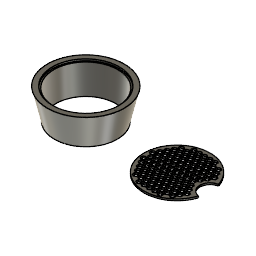
toyota-cup-holder (Autodesk Fusion 360 design; units mm, degrees)
part number: 2026-06-03-15-31-26-148
Autodesk Fusion 360 part; units mm, degrees
sketch "Sketch15" plane through (0, 0, 0) normal (0, 1, 0) x (1, 0, 0)
  line L0 (0, 0, 0) -> (0, 0, 40) construction
  line L1 (31, 0, 0) -> (37.8571, 0, 30)
  line L2 (37.8571, 0, 30) -> (32.8571, 0, 30)
  line L3 (32.8571, 0, 30) -> (32.8571, 0, 28.4)
  line L4 (32.8571, 0, 28.4) -> (31.4571, 0, 28.4)
  line L5 (31.4571, 0, 28.4) -> (29.8, 0, 0)
  line L6 (29.8, 0) -> (31, 0)
revolve "Revolve4" add sketch "Sketch15" angle 360 about axis through (0, 0, 0) along (0, 1, 0) contours L1 L2 L3 L4 L5 L6 in plane through (0, 0, 0) normal (0, 0, -1) makes body 1
move_body "Move1" bodies 1 to x (1, 0, 0) y (0, 0, 1) z (0, -1, 0) at (0, 0, 0)
sketch "Sketch16" plane through (0, 0, 0) normal (0, 0, 1) x (1, 0, 0)
  circle A0 centre (90, 0) radius 32.6
extrude "Extrude12" add sketch "Sketch16" along normal blind 1.6 separate body makes body 2
sketch "Sketch17" plane through (0, 0, 0) normal (0, 0, 1) x (1, 0, 0)
  circle A0 centre (122.6, 0) radius 10
extrude "Extrude13" cut sketch "Sketch17" along normal blind 1.6 bodies 2
sketch "HexGrid" plane through (0, 0, 0) normal (0, 0, 1) x (1, 0, 0)
  line L0 (81.6862, -25.8) -> (79.6077, -24.6)
  line L1 (79.6077, -24.6) -> (77.5292, -25.8)
  line L2 (77.5292, -25.8) -> (77.5292, -28.2)
  line L3 (77.5292, -28.2) -> (79.6077, -29.4)
  line L4 (79.6077, -29.4) -> (81.6862, -28.2)
  line L5 (81.6862, -28.2) -> (81.6862, -25.8)
  line L6 (86.8823, -25.8) -> (84.8038, -24.6)
  line L7 (84.8038, -24.6) -> (82.7254, -25.8)
  line L8 (82.7254, -25.8) -> (82.7254, -28.2)
  line L9 (82.7254, -28.2) -> (84.8038, -29.4)
  line L10 (84.8038, -29.4) -> (86.8823, -28.2)
  line L11 (86.8823, -28.2) -> (86.8823, -25.8)
  line L12 (92.0785, -25.8) -> (90, -24.6)
  line L13 (90, -24.6) -> (87.9215, -25.8)
  line L14 (87.9215, -25.8) -> (87.9215, -28.2)
  line L15 (87.9215, -28.2) -> (90, -29.4)
  line L16 (90, -29.4) -> (92.0785, -28.2)
  line L17 (92.0785, -28.2) -> (92.0785, -25.8)
  line L18 (97.2746, -25.8) -> (95.1962, -24.6)
  line L19 (95.1962, -24.6) -> (93.1177, -25.8)
  line L20 (93.1177, -25.8) -> (93.1177, -28.2)
  line L21 (93.1177, -28.2) -> (95.1962, -29.4)
  line L22 (95.1962, -29.4) -> (97.2746, -28.2)
  line L23 (97.2746, -28.2) -> (97.2746, -25.8)
  line L24 (102.4708, -25.8) -> (100.3923, -24.6)
  line L25 (100.3923, -24.6) -> (98.3138, -25.8)
  line L26 (98.3138, -25.8) -> (98.3138, -28.2)
  line L27 (98.3138, -28.2) -> (100.3923, -29.4)
  line L28 (100.3923, -29.4) -> (102.4708, -28.2)
  line L29 (102.4708, -28.2) -> (102.4708, -25.8)
  line L30 (73.8919, -21.3) -> (71.8135, -20.1)
  line L31 (71.8135, -20.1) -> (69.735, -21.3)
  line L32 (69.735, -21.3) -> (69.735, -23.7)
  line L33 (69.735, -23.7) -> (71.8135, -24.9)
  line L34 (71.8135, -24.9) -> (73.8919, -23.7)
  line L35 (73.8919, -23.7) -> (73.8919, -21.3)
  line L36 (79.0881, -21.3) -> (77.0096, -20.1)
  line L37 (77.0096, -20.1) -> (74.9312, -21.3)
  line L38 (74.9312, -21.3) -> (74.9312, -23.7)
  line L39 (74.9312, -23.7) -> (77.0096, -24.9)
  line L40 (77.0096, -24.9) -> (79.0881, -23.7)
  line L41 (79.0881, -23.7) -> (79.0881, -21.3)
  line L42 (84.2842, -21.3) -> (82.2058, -20.1)
  line L43 (82.2058, -20.1) -> (80.1273, -21.3)
  line L44 (80.1273, -21.3) -> (80.1273, -23.7)
  line L45 (80.1273, -23.7) -> (82.2058, -24.9)
  line L46 (82.2058, -24.9) -> (84.2842, -23.7)
  line L47 (84.2842, -23.7) -> (84.2842, -21.3)
  line L48 (89.4804, -21.3) -> (87.4019, -20.1)
  line L49 (87.4019, -20.1) -> (85.3235, -21.3)
  line L50 (85.3235, -21.3) -> (85.3235, -23.7)
  line L51 (85.3235, -23.7) -> (87.4019, -24.9)
  line L52 (87.4019, -24.9) -> (89.4804, -23.7)
  line L53 (89.4804, -23.7) -> (89.4804, -21.3)
  line L54 (94.6765, -21.3) -> (92.5981, -20.1)
  line L55 (92.5981, -20.1) -> (90.5196, -21.3)
  line L56 (90.5196, -21.3) -> (90.5196, -23.7)
  line L57 (90.5196, -23.7) -> (92.5981, -24.9)
  line L58 (92.5981, -24.9) -> (94.6765, -23.7)
  line L59 (94.6765, -23.7) -> (94.6765, -21.3)
  line L60 (99.8727, -21.3) -> (97.7942, -20.1)
  line L61 (97.7942, -20.1) -> (95.7158, -21.3)
  line L62 (95.7158, -21.3) -> (95.7158, -23.7)
  line L63 (95.7158, -23.7) -> (97.7942, -24.9)
  line L64 (97.7942, -24.9) -> (99.8727, -23.7)
  line L65 (99.8727, -23.7) -> (99.8727, -21.3)
  line L66 (105.0688, -21.3) -> (102.9904, -20.1)
  line L67 (102.9904, -20.1) -> (100.9119, -21.3)
  line L68 (100.9119, -21.3) -> (100.9119, -23.7)
  line L69 (100.9119, -23.7) -> (102.9904, -24.9)
  line L70 (102.9904, -24.9) -> (105.0688, -23.7)
  line L71 (105.0688, -23.7) -> (105.0688, -21.3)
  line L72 (110.265, -21.3) -> (108.1865, -20.1)
  line L73 (108.1865, -20.1) -> (106.1081, -21.3)
  line L74 (106.1081, -21.3) -> (106.1081, -23.7)
  line L75 (106.1081, -23.7) -> (108.1865, -24.9)
  line L76 (108.1865, -24.9) -> (110.265, -23.7)
  line L77 (110.265, -23.7) -> (110.265, -21.3)
  line L78 (71.2939, -16.8) -> (69.2154, -15.6)
  line L79 (69.2154, -15.6) -> (67.1369, -16.8)
  line L80 (67.1369, -16.8) -> (67.1369, -19.2)
  line L81 (67.1369, -19.2) -> (69.2154, -20.4)
  line L82 (69.2154, -20.4) -> (71.2939, -19.2)
  line L83 (71.2939, -19.2) -> (71.2939, -16.8)
  line L84 (76.49, -16.8) -> (74.4115, -15.6)
  line L85 (74.4115, -15.6) -> (72.3331, -16.8)
  line L86 (72.3331, -16.8) -> (72.3331, -19.2)
  line L87 (72.3331, -19.2) -> (74.4115, -20.4)
  line L88 (74.4115, -20.4) -> (76.49, -19.2)
  line L89 (76.49, -19.2) -> (76.49, -16.8)
  line L90 (81.6862, -16.8) -> (79.6077, -15.6)
  line L91 (79.6077, -15.6) -> (77.5292, -16.8)
  line L92 (77.5292, -16.8) -> (77.5292, -19.2)
  line L93 (77.5292, -19.2) -> (79.6077, -20.4)
  line L94 (79.6077, -20.4) -> (81.6862, -19.2)
  line L95 (81.6862, -19.2) -> (81.6862, -16.8)
  line L96 (86.8823, -16.8) -> (84.8038, -15.6)
  line L97 (84.8038, -15.6) -> (82.7254, -16.8)
  line L98 (82.7254, -16.8) -> (82.7254, -19.2)
  line L99 (82.7254, -19.2) -> (84.8038, -20.4)
  line L100 (84.8038, -20.4) -> (86.8823, -19.2)
  line L101 (86.8823, -19.2) -> (86.8823, -16.8)
  line L102 (92.0785, -16.8) -> (90, -15.6)
  line L103 (90, -15.6) -> (87.9215, -16.8)
  line L104 (87.9215, -16.8) -> (87.9215, -19.2)
  line L105 (87.9215, -19.2) -> (90, -20.4)
  line L106 (90, -20.4) -> (92.0785, -19.2)
  line L107 (92.0785, -19.2) -> (92.0785, -16.8)
  line L108 (97.2746, -16.8) -> (95.1962, -15.6)
  line L109 (95.1962, -15.6) -> (93.1177, -16.8)
  line L110 (93.1177, -16.8) -> (93.1177, -19.2)
  line L111 (93.1177, -19.2) -> (95.1962, -20.4)
  line L112 (95.1962, -20.4) -> (97.2746, -19.2)
  line L113 (97.2746, -19.2) -> (97.2746, -16.8)
  line L114 (102.4708, -16.8) -> (100.3923, -15.6)
  line L115 (100.3923, -15.6) -> (98.3138, -16.8)
  line L116 (98.3138, -16.8) -> (98.3138, -19.2)
  line L117 (98.3138, -19.2) -> (100.3923, -20.4)
  line L118 (100.3923, -20.4) -> (102.4708, -19.2)
  line L119 (102.4708, -19.2) -> (102.4708, -16.8)
  line L120 (107.6669, -16.8) -> (105.5885, -15.6)
  line L121 (105.5885, -15.6) -> (103.51, -16.8)
  line L122 (103.51, -16.8) -> (103.51, -19.2)
  line L123 (103.51, -19.2) -> (105.5885, -20.4)
  line L124 (105.5885, -20.4) -> (107.6669, -19.2)
  line L125 (107.6669, -19.2) -> (107.6669, -16.8)
  line L126 (112.8631, -16.8) -> (110.7846, -15.6)
  line L127 (110.7846, -15.6) -> (108.7061, -16.8)
  line L128 (108.7061, -16.8) -> (108.7061, -19.2)
  line L129 (108.7061, -19.2) -> (110.7846, -20.4)
  line L130 (110.7846, -20.4) -> (112.8631, -19.2)
  line L131 (112.8631, -19.2) -> (112.8631, -16.8)
  line L132 (68.6958, -12.3) -> (66.6173, -11.1)
  line L133 (66.6173, -11.1) -> (64.5389, -12.3)
  line L134 (64.5389, -12.3) -> (64.5389, -14.7)
  line L135 (64.5389, -14.7) -> (66.6173, -15.9)
  line L136 (66.6173, -15.9) -> (68.6958, -14.7)
  line L137 (68.6958, -14.7) -> (68.6958, -12.3)
  line L138 (73.8919, -12.3) -> (71.8135, -11.1)
  line L139 (71.8135, -11.1) -> (69.735, -12.3)
  line L140 (69.735, -12.3) -> (69.735, -14.7)
  line L141 (69.735, -14.7) -> (71.8135, -15.9)
  line L142 (71.8135, -15.9) -> (73.8919, -14.7)
  line L143 (73.8919, -14.7) -> (73.8919, -12.3)
  line L144 (79.0881, -12.3) -> (77.0096, -11.1)
  line L145 (77.0096, -11.1) -> (74.9312, -12.3)
  line L146 (74.9312, -12.3) -> (74.9312, -14.7)
  line L147 (74.9312, -14.7) -> (77.0096, -15.9)
  line L148 (77.0096, -15.9) -> (79.0881, -14.7)
  line L149 (79.0881, -14.7) -> (79.0881, -12.3)
  line L150 (84.2842, -12.3) -> (82.2058, -11.1)
  line L151 (82.2058, -11.1) -> (80.1273, -12.3)
  line L152 (80.1273, -12.3) -> (80.1273, -14.7)
  line L153 (80.1273, -14.7) -> (82.2058, -15.9)
  line L154 (82.2058, -15.9) -> (84.2842, -14.7)
  line L155 (84.2842, -14.7) -> (84.2842, -12.3)
  line L156 (89.4804, -12.3) -> (87.4019, -11.1)
  line L157 (87.4019, -11.1) -> (85.3235, -12.3)
  line L158 (85.3235, -12.3) -> (85.3235, -14.7)
  line L159 (85.3235, -14.7) -> (87.4019, -15.9)
  line L160 (87.4019, -15.9) -> (89.4804, -14.7)
  line L161 (89.4804, -14.7) -> (89.4804, -12.3)
  line L162 (94.6765, -12.3) -> (92.5981, -11.1)
  line L163 (92.5981, -11.1) -> (90.5196, -12.3)
  line L164 (90.5196, -12.3) -> (90.5196, -14.7)
  line L165 (90.5196, -14.7) -> (92.5981, -15.9)
  line L166 (92.5981, -15.9) -> (94.6765, -14.7)
  line L167 (94.6765, -14.7) -> (94.6765, -12.3)
  line L168 (99.8727, -12.3) -> (97.7942, -11.1)
  line L169 (97.7942, -11.1) -> (95.7158, -12.3)
  line L170 (95.7158, -12.3) -> (95.7158, -14.7)
  line L171 (95.7158, -14.7) -> (97.7942, -15.9)
  line L172 (97.7942, -15.9) -> (99.8727, -14.7)
  line L173 (99.8727, -14.7) -> (99.8727, -12.3)
  line L174 (105.0688, -12.3) -> (102.9904, -11.1)
  line L175 (102.9904, -11.1) -> (100.9119, -12.3)
  line L176 (100.9119, -12.3) -> (100.9119, -14.7)
  line L177 (100.9119, -14.7) -> (102.9904, -15.9)
  line L178 (102.9904, -15.9) -> (105.0688, -14.7)
  line L179 (105.0688, -14.7) -> (105.0688, -12.3)
  line L180 (110.265, -12.3) -> (108.1865, -11.1)
  line L181 (108.1865, -11.1) -> (106.1081, -12.3)
  line L182 (106.1081, -12.3) -> (106.1081, -14.7)
  line L183 (106.1081, -14.7) -> (108.1865, -15.9)
  line L184 (108.1865, -15.9) -> (110.265, -14.7)
  line L185 (110.265, -14.7) -> (110.265, -12.3)
  line L186 (115.4611, -12.3) -> (113.3827, -11.1)
  line L187 (113.3827, -11.1) -> (111.3042, -12.3)
  line L188 (111.3042, -12.3) -> (111.3042, -14.7)
  line L189 (111.3042, -14.7) -> (113.3827, -15.9)
  line L190 (113.3827, -15.9) -> (115.4611, -14.7)
  line L191 (115.4611, -14.7) -> (115.4611, -12.3)
  line L192 (66.0977, -7.8) -> (64.0192, -6.6)
  line L193 (64.0192, -6.6) -> (61.9408, -7.8)
  line L194 (61.9408, -7.8) -> (61.9408, -10.2)
  line L195 (61.9408, -10.2) -> (64.0192, -11.4)
  line L196 (64.0192, -11.4) -> (66.0977, -10.2)
  line L197 (66.0977, -10.2) -> (66.0977, -7.8)
  line L198 (71.2939, -7.8) -> (69.2154, -6.6)
  line L199 (69.2154, -6.6) -> (67.1369, -7.8)
  line L200 (67.1369, -7.8) -> (67.1369, -10.2)
  line L201 (67.1369, -10.2) -> (69.2154, -11.4)
  line L202 (69.2154, -11.4) -> (71.2939, -10.2)
  line L203 (71.2939, -10.2) -> (71.2939, -7.8)
  line L204 (76.49, -7.8) -> (74.4115, -6.6)
  line L205 (74.4115, -6.6) -> (72.3331, -7.8)
  line L206 (72.3331, -7.8) -> (72.3331, -10.2)
  line L207 (72.3331, -10.2) -> (74.4115, -11.4)
  line L208 (74.4115, -11.4) -> (76.49, -10.2)
  line L209 (76.49, -10.2) -> (76.49, -7.8)
  line L210 (81.6862, -7.8) -> (79.6077, -6.6)
  line L211 (79.6077, -6.6) -> (77.5292, -7.8)
  line L212 (77.5292, -7.8) -> (77.5292, -10.2)
  line L213 (77.5292, -10.2) -> (79.6077, -11.4)
  line L214 (79.6077, -11.4) -> (81.6862, -10.2)
  line L215 (81.6862, -10.2) -> (81.6862, -7.8)
  line L216 (86.8823, -7.8) -> (84.8038, -6.6)
  line L217 (84.8038, -6.6) -> (82.7254, -7.8)
  line L218 (82.7254, -7.8) -> (82.7254, -10.2)
  line L219 (82.7254, -10.2) -> (84.8038, -11.4)
  line L220 (84.8038, -11.4) -> (86.8823, -10.2)
  line L221 (86.8823, -10.2) -> (86.8823, -7.8)
  line L222 (92.0785, -7.8) -> (90, -6.6)
  line L223 (90, -6.6) -> (87.9215, -7.8)
  line L224 (87.9215, -7.8) -> (87.9215, -10.2)
  line L225 (87.9215, -10.2) -> (90, -11.4)
  line L226 (90, -11.4) -> (92.0785, -10.2)
  line L227 (92.0785, -10.2) -> (92.0785, -7.8)
  line L228 (97.2746, -7.8) -> (95.1962, -6.6)
  line L229 (95.1962, -6.6) -> (93.1177, -7.8)
  line L230 (93.1177, -7.8) -> (93.1177, -10.2)
  line L231 (93.1177, -10.2) -> (95.1962, -11.4)
  line L232 (95.1962, -11.4) -> (97.2746, -10.2)
  line L233 (97.2746, -10.2) -> (97.2746, -7.8)
  line L234 (102.4708, -7.8) -> (100.3923, -6.6)
  line L235 (100.3923, -6.6) -> (98.3138, -7.8)
  line L236 (98.3138, -7.8) -> (98.3138, -10.2)
  line L237 (98.3138, -10.2) -> (100.3923, -11.4)
  line L238 (100.3923, -11.4) -> (102.4708, -10.2)
  line L239 (102.4708, -10.2) -> (102.4708, -7.8)
  line L240 (107.6669, -7.8) -> (105.5885, -6.6)
  line L241 (105.5885, -6.6) -> (103.51, -7.8)
  line L242 (103.51, -7.8) -> (103.51, -10.2)
  line L243 (103.51, -10.2) -> (105.5885, -11.4)
  line L244 (105.5885, -11.4) -> (107.6669, -10.2)
  line L245 (107.6669, -10.2) -> (107.6669, -7.8)
  line L246 (112.8631, -7.8) -> (110.7846, -6.6)
  line L247 (110.7846, -6.6) -> (108.7061, -7.8)
  line L248 (108.7061, -7.8) -> (108.7061, -10.2)
  line L249 (108.7061, -10.2) -> (110.7846, -11.4)
  line L250 (110.7846, -11.4) -> (112.8631, -10.2)
  line L251 (112.8631, -10.2) -> (112.8631, -7.8)
  line L252 (63.4996, -3.3) -> (61.4212, -2.1)
  line L253 (61.4212, -2.1) -> (59.3427, -3.3)
  line L254 (59.3427, -3.3) -> (59.3427, -5.7)
  line L255 (59.3427, -5.7) -> (61.4212, -6.9)
  line L256 (61.4212, -6.9) -> (63.4996, -5.7)
  line L257 (63.4996, -5.7) -> (63.4996, -3.3)
  line L258 (68.6958, -3.3) -> (66.6173, -2.1)
  line L259 (66.6173, -2.1) -> (64.5389, -3.3)
  line L260 (64.5389, -3.3) -> (64.5389, -5.7)
  line L261 (64.5389, -5.7) -> (66.6173, -6.9)
  line L262 (66.6173, -6.9) -> (68.6958, -5.7)
  line L263 (68.6958, -5.7) -> (68.6958, -3.3)
  line L264 (73.8919, -3.3) -> (71.8135, -2.1)
  line L265 (71.8135, -2.1) -> (69.735, -3.3)
  line L266 (69.735, -3.3) -> (69.735, -5.7)
  line L267 (69.735, -5.7) -> (71.8135, -6.9)
  line L268 (71.8135, -6.9) -> (73.8919, -5.7)
  line L269 (73.8919, -5.7) -> (73.8919, -3.3)
  line L270 (79.0881, -3.3) -> (77.0096, -2.1)
  line L271 (77.0096, -2.1) -> (74.9312, -3.3)
  line L272 (74.9312, -3.3) -> (74.9312, -5.7)
  line L273 (74.9312, -5.7) -> (77.0096, -6.9)
  line L274 (77.0096, -6.9) -> (79.0881, -5.7)
  line L275 (79.0881, -5.7) -> (79.0881, -3.3)
  line L276 (84.2842, -3.3) -> (82.2058, -2.1)
  line L277 (82.2058, -2.1) -> (80.1273, -3.3)
  line L278 (80.1273, -3.3) -> (80.1273, -5.7)
  line L279 (80.1273, -5.7) -> (82.2058, -6.9)
  line L280 (82.2058, -6.9) -> (84.2842, -5.7)
  line L281 (84.2842, -5.7) -> (84.2842, -3.3)
  line L282 (89.4804, -3.3) -> (87.4019, -2.1)
  line L283 (87.4019, -2.1) -> (85.3235, -3.3)
  line L284 (85.3235, -3.3) -> (85.3235, -5.7)
  line L285 (85.3235, -5.7) -> (87.4019, -6.9)
  line L286 (87.4019, -6.9) -> (89.4804, -5.7)
  line L287 (89.4804, -5.7) -> (89.4804, -3.3)
  line L288 (94.6765, -3.3) -> (92.5981, -2.1)
  line L289 (92.5981, -2.1) -> (90.5196, -3.3)
  line L290 (90.5196, -3.3) -> (90.5196, -5.7)
  line L291 (90.5196, -5.7) -> (92.5981, -6.9)
  line L292 (92.5981, -6.9) -> (94.6765, -5.7)
  line L293 (94.6765, -5.7) -> (94.6765, -3.3)
  line L294 (99.8727, -3.3) -> (97.7942, -2.1)
  line L295 (97.7942, -2.1) -> (95.7158, -3.3)
  line L296 (95.7158, -3.3) -> (95.7158, -5.7)
  line L297 (95.7158, -5.7) -> (97.7942, -6.9)
  line L298 (97.7942, -6.9) -> (99.8727, -5.7)
  line L299 (99.8727, -5.7) -> (99.8727, -3.3)
  line L300 (105.0688, -3.3) -> (102.9904, -2.1)
  line L301 (102.9904, -2.1) -> (100.9119, -3.3)
  line L302 (100.9119, -3.3) -> (100.9119, -5.7)
  line L303 (100.9119, -5.7) -> (102.9904, -6.9)
  line L304 (102.9904, -6.9) -> (105.0688, -5.7)
  line L305 (105.0688, -5.7) -> (105.0688, -3.3)
  line L306 (110.265, -3.3) -> (108.1865, -2.1)
  line L307 (108.1865, -2.1) -> (106.1081, -3.3)
  line L308 (106.1081, -3.3) -> (106.1081, -5.7)
  line L309 (106.1081, -5.7) -> (108.1865, -6.9)
  line L310 (108.1865, -6.9) -> (110.265, -5.7)
  line L311 (110.265, -5.7) -> (110.265, -3.3)
  line L312 (66.0977, 1.2) -> (64.0192, 2.4)
  line L313 (64.0192, 2.4) -> (61.9408, 1.2)
  line L314 (61.9408, 1.2) -> (61.9408, -1.2)
  line L315 (61.9408, -1.2) -> (64.0192, -2.4)
  line L316 (64.0192, -2.4) -> (66.0977, -1.2)
  line L317 (66.0977, -1.2) -> (66.0977, 1.2)
  line L318 (71.2939, 1.2) -> (69.2154, 2.4)
  line L319 (69.2154, 2.4) -> (67.1369, 1.2)
  line L320 (67.1369, 1.2) -> (67.1369, -1.2)
  line L321 (67.1369, -1.2) -> (69.2154, -2.4)
  line L322 (69.2154, -2.4) -> (71.2939, -1.2)
  line L323 (71.2939, -1.2) -> (71.2939, 1.2)
  line L324 (76.49, 1.2) -> (74.4115, 2.4)
  line L325 (74.4115, 2.4) -> (72.3331, 1.2)
  line L326 (72.3331, 1.2) -> (72.3331, -1.2)
  line L327 (72.3331, -1.2) -> (74.4115, -2.4)
  line L328 (74.4115, -2.4) -> (76.49, -1.2)
  line L329 (76.49, -1.2) -> (76.49, 1.2)
  line L330 (81.6862, 1.2) -> (79.6077, 2.4)
  line L331 (79.6077, 2.4) -> (77.5292, 1.2)
  line L332 (77.5292, 1.2) -> (77.5292, -1.2)
  line L333 (77.5292, -1.2) -> (79.6077, -2.4)
  line L334 (79.6077, -2.4) -> (81.6862, -1.2)
  line L335 (81.6862, -1.2) -> (81.6862, 1.2)
  line L336 (86.8823, 1.2) -> (84.8038, 2.4)
  line L337 (84.8038, 2.4) -> (82.7254, 1.2)
  line L338 (82.7254, 1.2) -> (82.7254, -1.2)
  line L339 (82.7254, -1.2) -> (84.8038, -2.4)
  line L340 (84.8038, -2.4) -> (86.8823, -1.2)
  line L341 (86.8823, -1.2) -> (86.8823, 1.2)
  line L342 (92.0785, 1.2) -> (90, 2.4)
  line L343 (90, 2.4) -> (87.9215, 1.2)
  line L344 (87.9215, 1.2) -> (87.9215, -1.2)
  line L345 (87.9215, -1.2) -> (90, -2.4)
  line L346 (90, -2.4) -> (92.0785, -1.2)
  line L347 (92.0785, -1.2) -> (92.0785, 1.2)
  line L348 (97.2746, 1.2) -> (95.1962, 2.4)
  line L349 (95.1962, 2.4) -> (93.1177, 1.2)
  line L350 (93.1177, 1.2) -> (93.1177, -1.2)
  line L351 (93.1177, -1.2) -> (95.1962, -2.4)
  line L352 (95.1962, -2.4) -> (97.2746, -1.2)
  line L353 (97.2746, -1.2) -> (97.2746, 1.2)
  line L354 (102.4708, 1.2) -> (100.3923, 2.4)
  line L355 (100.3923, 2.4) -> (98.3138, 1.2)
  line L356 (98.3138, 1.2) -> (98.3138, -1.2)
  line L357 (98.3138, -1.2) -> (100.3923, -2.4)
  line L358 (100.3923, -2.4) -> (102.4708, -1.2)
  line L359 (102.4708, -1.2) -> (102.4708, 1.2)
  line L360 (107.6669, 1.2) -> (105.5885, 2.4)
  line L361 (105.5885, 2.4) -> (103.51, 1.2)
  line L362 (103.51, 1.2) -> (103.51, -1.2)
  line L363 (103.51, -1.2) -> (105.5885, -2.4)
  line L364 (105.5885, -2.4) -> (107.6669, -1.2)
  line L365 (107.6669, -1.2) -> (107.6669, 1.2)
  line L366 (63.4996, 5.7) -> (61.4212, 6.9)
  line L367 (61.4212, 6.9) -> (59.3427, 5.7)
  line L368 (59.3427, 5.7) -> (59.3427, 3.3)
  line L369 (59.3427, 3.3) -> (61.4212, 2.1)
  line L370 (61.4212, 2.1) -> (63.4996, 3.3)
  line L371 (63.4996, 3.3) -> (63.4996, 5.7)
  line L372 (68.6958, 5.7) -> (66.6173, 6.9)
  line L373 (66.6173, 6.9) -> (64.5389, 5.7)
  line L374 (64.5389, 5.7) -> (64.5389, 3.3)
  line L375 (64.5389, 3.3) -> (66.6173, 2.1)
  line L376 (66.6173, 2.1) -> (68.6958, 3.3)
  line L377 (68.6958, 3.3) -> (68.6958, 5.7)
  line L378 (73.8919, 5.7) -> (71.8135, 6.9)
  line L379 (71.8135, 6.9) -> (69.735, 5.7)
  line L380 (69.735, 5.7) -> (69.735, 3.3)
  line L381 (69.735, 3.3) -> (71.8135, 2.1)
  line L382 (71.8135, 2.1) -> (73.8919, 3.3)
  line L383 (73.8919, 3.3) -> (73.8919, 5.7)
  line L384 (79.0881, 5.7) -> (77.0096, 6.9)
  line L385 (77.0096, 6.9) -> (74.9312, 5.7)
  line L386 (74.9312, 5.7) -> (74.9312, 3.3)
  line L387 (74.9312, 3.3) -> (77.0096, 2.1)
  line L388 (77.0096, 2.1) -> (79.0881, 3.3)
  line L389 (79.0881, 3.3) -> (79.0881, 5.7)
  line L390 (84.2842, 5.7) -> (82.2058, 6.9)
  line L391 (82.2058, 6.9) -> (80.1273, 5.7)
  line L392 (80.1273, 5.7) -> (80.1273, 3.3)
  line L393 (80.1273, 3.3) -> (82.2058, 2.1)
  line L394 (82.2058, 2.1) -> (84.2842, 3.3)
  line L395 (84.2842, 3.3) -> (84.2842, 5.7)
  line L396 (89.4804, 5.7) -> (87.4019, 6.9)
  line L397 (87.4019, 6.9) -> (85.3235, 5.7)
  line L398 (85.3235, 5.7) -> (85.3235, 3.3)
  line L399 (85.3235, 3.3) -> (87.4019, 2.1)
  line L400 (87.4019, 2.1) -> (89.4804, 3.3)
  line L401 (89.4804, 3.3) -> (89.4804, 5.7)
  line L402 (94.6765, 5.7) -> (92.5981, 6.9)
  line L403 (92.5981, 6.9) -> (90.5196, 5.7)
  line L404 (90.5196, 5.7) -> (90.5196, 3.3)
  line L405 (90.5196, 3.3) -> (92.5981, 2.1)
  line L406 (92.5981, 2.1) -> (94.6765, 3.3)
  line L407 (94.6765, 3.3) -> (94.6765, 5.7)
  line L408 (99.8727, 5.7) -> (97.7942, 6.9)
  line L409 (97.7942, 6.9) -> (95.7158, 5.7)
  line L410 (95.7158, 5.7) -> (95.7158, 3.3)
  line L411 (95.7158, 3.3) -> (97.7942, 2.1)
  line L412 (97.7942, 2.1) -> (99.8727, 3.3)
  line L413 (99.8727, 3.3) -> (99.8727, 5.7)
  line L414 (105.0688, 5.7) -> (102.9904, 6.9)
  line L415 (102.9904, 6.9) -> (100.9119, 5.7)
  line L416 (100.9119, 5.7) -> (100.9119, 3.3)
  line L417 (100.9119, 3.3) -> (102.9904, 2.1)
  line L418 (102.9904, 2.1) -> (105.0688, 3.3)
  line L419 (105.0688, 3.3) -> (105.0688, 5.7)
  line L420 (110.265, 5.7) -> (108.1865, 6.9)
  line L421 (108.1865, 6.9) -> (106.1081, 5.7)
  line L422 (106.1081, 5.7) -> (106.1081, 3.3)
  line L423 (106.1081, 3.3) -> (108.1865, 2.1)
  line L424 (108.1865, 2.1) -> (110.265, 3.3)
  line L425 (110.265, 3.3) -> (110.265, 5.7)
  line L426 (66.0977, 10.2) -> (64.0192, 11.4)
  line L427 (64.0192, 11.4) -> (61.9408, 10.2)
  line L428 (61.9408, 10.2) -> (61.9408, 7.8)
  line L429 (61.9408, 7.8) -> (64.0192, 6.6)
  line L430 (64.0192, 6.6) -> (66.0977, 7.8)
  line L431 (66.0977, 7.8) -> (66.0977, 10.2)
  line L432 (71.2939, 10.2) -> (69.2154, 11.4)
  line L433 (69.2154, 11.4) -> (67.1369, 10.2)
  line L434 (67.1369, 10.2) -> (67.1369, 7.8)
  line L435 (67.1369, 7.8) -> (69.2154, 6.6)
  line L436 (69.2154, 6.6) -> (71.2939, 7.8)
  line L437 (71.2939, 7.8) -> (71.2939, 10.2)
  line L438 (76.49, 10.2) -> (74.4115, 11.4)
  line L439 (74.4115, 11.4) -> (72.3331, 10.2)
  line L440 (72.3331, 10.2) -> (72.3331, 7.8)
  line L441 (72.3331, 7.8) -> (74.4115, 6.6)
  line L442 (74.4115, 6.6) -> (76.49, 7.8)
  line L443 (76.49, 7.8) -> (76.49, 10.2)
  line L444 (81.6862, 10.2) -> (79.6077, 11.4)
  line L445 (79.6077, 11.4) -> (77.5292, 10.2)
  line L446 (77.5292, 10.2) -> (77.5292, 7.8)
  line L447 (77.5292, 7.8) -> (79.6077, 6.6)
  line L448 (79.6077, 6.6) -> (81.6862, 7.8)
  line L449 (81.6862, 7.8) -> (81.6862, 10.2)
  line L450 (86.8823, 10.2) -> (84.8038, 11.4)
  line L451 (84.8038, 11.4) -> (82.7254, 10.2)
  line L452 (82.7254, 10.2) -> (82.7254, 7.8)
  line L453 (82.7254, 7.8) -> (84.8038, 6.6)
  line L454 (84.8038, 6.6) -> (86.8823, 7.8)
  line L455 (86.8823, 7.8) -> (86.8823, 10.2)
  line L456 (92.0785, 10.2) -> (90, 11.4)
  line L457 (90, 11.4) -> (87.9215, 10.2)
  line L458 (87.9215, 10.2) -> (87.9215, 7.8)
  line L459 (87.9215, 7.8) -> (90, 6.6)
  line L460 (90, 6.6) -> (92.0785, 7.8)
  line L461 (92.0785, 7.8) -> (92.0785, 10.2)
  line L462 (97.2746, 10.2) -> (95.1962, 11.4)
  line L463 (95.1962, 11.4) -> (93.1177, 10.2)
  line L464 (93.1177, 10.2) -> (93.1177, 7.8)
  line L465 (93.1177, 7.8) -> (95.1962, 6.6)
  line L466 (95.1962, 6.6) -> (97.2746, 7.8)
  line L467 (97.2746, 7.8) -> (97.2746, 10.2)
  line L468 (102.4708, 10.2) -> (100.3923, 11.4)
  line L469 (100.3923, 11.4) -> (98.3138, 10.2)
  line L470 (98.3138, 10.2) -> (98.3138, 7.8)
  line L471 (98.3138, 7.8) -> (100.3923, 6.6)
  line L472 (100.3923, 6.6) -> (102.4708, 7.8)
  line L473 (102.4708, 7.8) -> (102.4708, 10.2)
  line L474 (107.6669, 10.2) -> (105.5885, 11.4)
  line L475 (105.5885, 11.4) -> (103.51, 10.2)
  line L476 (103.51, 10.2) -> (103.51, 7.8)
  line L477 (103.51, 7.8) -> (105.5885, 6.6)
  line L478 (105.5885, 6.6) -> (107.6669, 7.8)
  line L479 (107.6669, 7.8) -> (107.6669, 10.2)
  line L480 (112.8631, 10.2) -> (110.7846, 11.4)
  line L481 (110.7846, 11.4) -> (108.7061, 10.2)
  line L482 (108.7061, 10.2) -> (108.7061, 7.8)
  line L483 (108.7061, 7.8) -> (110.7846, 6.6)
  line L484 (110.7846, 6.6) -> (112.8631, 7.8)
  line L485 (112.8631, 7.8) -> (112.8631, 10.2)
  line L486 (68.6958, 14.7) -> (66.6173, 15.9)
  line L487 (66.6173, 15.9) -> (64.5389, 14.7)
  line L488 (64.5389, 14.7) -> (64.5389, 12.3)
  line L489 (64.5389, 12.3) -> (66.6173, 11.1)
  line L490 (66.6173, 11.1) -> (68.6958, 12.3)
  line L491 (68.6958, 12.3) -> (68.6958, 14.7)
  line L492 (73.8919, 14.7) -> (71.8135, 15.9)
  line L493 (71.8135, 15.9) -> (69.735, 14.7)
  line L494 (69.735, 14.7) -> (69.735, 12.3)
  line L495 (69.735, 12.3) -> (71.8135, 11.1)
  line L496 (71.8135, 11.1) -> (73.8919, 12.3)
  line L497 (73.8919, 12.3) -> (73.8919, 14.7)
  line L498 (79.0881, 14.7) -> (77.0096, 15.9)
  line L499 (77.0096, 15.9) -> (74.9312, 14.7)
  line L500 (74.9312, 14.7) -> (74.9312, 12.3)
  line L501 (74.9312, 12.3) -> (77.0096, 11.1)
  line L502 (77.0096, 11.1) -> (79.0881, 12.3)
  line L503 (79.0881, 12.3) -> (79.0881, 14.7)
  line L504 (84.2842, 14.7) -> (82.2058, 15.9)
  line L505 (82.2058, 15.9) -> (80.1273, 14.7)
  line L506 (80.1273, 14.7) -> (80.1273, 12.3)
  line L507 (80.1273, 12.3) -> (82.2058, 11.1)
  line L508 (82.2058, 11.1) -> (84.2842, 12.3)
  line L509 (84.2842, 12.3) -> (84.2842, 14.7)
  line L510 (89.4804, 14.7) -> (87.4019, 15.9)
  line L511 (87.4019, 15.9) -> (85.3235, 14.7)
  line L512 (85.3235, 14.7) -> (85.3235, 12.3)
  line L513 (85.3235, 12.3) -> (87.4019, 11.1)
  line L514 (87.4019, 11.1) -> (89.4804, 12.3)
  line L515 (89.4804, 12.3) -> (89.4804, 14.7)
  line L516 (94.6765, 14.7) -> (92.5981, 15.9)
  line L517 (92.5981, 15.9) -> (90.5196, 14.7)
  line L518 (90.5196, 14.7) -> (90.5196, 12.3)
  line L519 (90.5196, 12.3) -> (92.5981, 11.1)
  line L520 (92.5981, 11.1) -> (94.6765, 12.3)
  line L521 (94.6765, 12.3) -> (94.6765, 14.7)
  line L522 (99.8727, 14.7) -> (97.7942, 15.9)
  line L523 (97.7942, 15.9) -> (95.7158, 14.7)
  line L524 (95.7158, 14.7) -> (95.7158, 12.3)
  line L525 (95.7158, 12.3) -> (97.7942, 11.1)
  line L526 (97.7942, 11.1) -> (99.8727, 12.3)
  line L527 (99.8727, 12.3) -> (99.8727, 14.7)
  line L528 (105.0688, 14.7) -> (102.9904, 15.9)
  line L529 (102.9904, 15.9) -> (100.9119, 14.7)
  line L530 (100.9119, 14.7) -> (100.9119, 12.3)
  line L531 (100.9119, 12.3) -> (102.9904, 11.1)
  line L532 (102.9904, 11.1) -> (105.0688, 12.3)
  line L533 (105.0688, 12.3) -> (105.0688, 14.7)
  line L534 (110.265, 14.7) -> (108.1865, 15.9)
  line L535 (108.1865, 15.9) -> (106.1081, 14.7)
  line L536 (106.1081, 14.7) -> (106.1081, 12.3)
  line L537 (106.1081, 12.3) -> (108.1865, 11.1)
  line L538 (108.1865, 11.1) -> (110.265, 12.3)
  line L539 (110.265, 12.3) -> (110.265, 14.7)
  line L540 (115.4611, 14.7) -> (113.3827, 15.9)
  line L541 (113.3827, 15.9) -> (111.3042, 14.7)
  line L542 (111.3042, 14.7) -> (111.3042, 12.3)
  line L543 (111.3042, 12.3) -> (113.3827, 11.1)
  line L544 (113.3827, 11.1) -> (115.4611, 12.3)
  line L545 (115.4611, 12.3) -> (115.4611, 14.7)
  line L546 (71.2939, 19.2) -> (69.2154, 20.4)
  line L547 (69.2154, 20.4) -> (67.1369, 19.2)
  line L548 (67.1369, 19.2) -> (67.1369, 16.8)
  line L549 (67.1369, 16.8) -> (69.2154, 15.6)
  line L550 (69.2154, 15.6) -> (71.2939, 16.8)
  line L551 (71.2939, 16.8) -> (71.2939, 19.2)
  line L552 (76.49, 19.2) -> (74.4115, 20.4)
  line L553 (74.4115, 20.4) -> (72.3331, 19.2)
  line L554 (72.3331, 19.2) -> (72.3331, 16.8)
  line L555 (72.3331, 16.8) -> (74.4115, 15.6)
  line L556 (74.4115, 15.6) -> (76.49, 16.8)
  line L557 (76.49, 16.8) -> (76.49, 19.2)
  line L558 (81.6862, 19.2) -> (79.6077, 20.4)
  line L559 (79.6077, 20.4) -> (77.5292, 19.2)
  line L560 (77.5292, 19.2) -> (77.5292, 16.8)
  line L561 (77.5292, 16.8) -> (79.6077, 15.6)
  line L562 (79.6077, 15.6) -> (81.6862, 16.8)
  line L563 (81.6862, 16.8) -> (81.6862, 19.2)
  line L564 (86.8823, 19.2) -> (84.8038, 20.4)
  line L565 (84.8038, 20.4) -> (82.7254, 19.2)
  line L566 (82.7254, 19.2) -> (82.7254, 16.8)
  line L567 (82.7254, 16.8) -> (84.8038, 15.6)
  line L568 (84.8038, 15.6) -> (86.8823, 16.8)
  line L569 (86.8823, 16.8) -> (86.8823, 19.2)
  line L570 (92.0785, 19.2) -> (90, 20.4)
  line L571 (90, 20.4) -> (87.9215, 19.2)
  line L572 (87.9215, 19.2) -> (87.9215, 16.8)
  line L573 (87.9215, 16.8) -> (90, 15.6)
  line L574 (90, 15.6) -> (92.0785, 16.8)
  line L575 (92.0785, 16.8) -> (92.0785, 19.2)
  line L576 (97.2746, 19.2) -> (95.1962, 20.4)
  line L577 (95.1962, 20.4) -> (93.1177, 19.2)
  line L578 (93.1177, 19.2) -> (93.1177, 16.8)
  line L579 (93.1177, 16.8) -> (95.1962, 15.6)
  line L580 (95.1962, 15.6) -> (97.2746, 16.8)
  line L581 (97.2746, 16.8) -> (97.2746, 19.2)
  line L582 (102.4708, 19.2) -> (100.3923, 20.4)
  line L583 (100.3923, 20.4) -> (98.3138, 19.2)
  line L584 (98.3138, 19.2) -> (98.3138, 16.8)
  line L585 (98.3138, 16.8) -> (100.3923, 15.6)
  line L586 (100.3923, 15.6) -> (102.4708, 16.8)
  line L587 (102.4708, 16.8) -> (102.4708, 19.2)
  line L588 (107.6669, 19.2) -> (105.5885, 20.4)
  line L589 (105.5885, 20.4) -> (103.51, 19.2)
  line L590 (103.51, 19.2) -> (103.51, 16.8)
  line L591 (103.51, 16.8) -> (105.5885, 15.6)
  line L592 (105.5885, 15.6) -> (107.6669, 16.8)
  line L593 (107.6669, 16.8) -> (107.6669, 19.2)
  line L594 (112.8631, 19.2) -> (110.7846, 20.4)
  line L595 (110.7846, 20.4) -> (108.7061, 19.2)
  line L596 (108.7061, 19.2) -> (108.7061, 16.8)
  line L597 (108.7061, 16.8) -> (110.7846, 15.6)
  line L598 (110.7846, 15.6) -> (112.8631, 16.8)
  line L599 (112.8631, 16.8) -> (112.8631, 19.2)
  line L600 (73.8919, 23.7) -> (71.8135, 24.9)
  line L601 (71.8135, 24.9) -> (69.735, 23.7)
  line L602 (69.735, 23.7) -> (69.735, 21.3)
  line L603 (69.735, 21.3) -> (71.8135, 20.1)
  line L604 (71.8135, 20.1) -> (73.8919, 21.3)
  line L605 (73.8919, 21.3) -> (73.8919, 23.7)
  line L606 (79.0881, 23.7) -> (77.0096, 24.9)
  line L607 (77.0096, 24.9) -> (74.9312, 23.7)
  line L608 (74.9312, 23.7) -> (74.9312, 21.3)
  line L609 (74.9312, 21.3) -> (77.0096, 20.1)
  line L610 (77.0096, 20.1) -> (79.0881, 21.3)
  line L611 (79.0881, 21.3) -> (79.0881, 23.7)
  line L612 (84.2842, 23.7) -> (82.2058, 24.9)
  line L613 (82.2058, 24.9) -> (80.1273, 23.7)
  line L614 (80.1273, 23.7) -> (80.1273, 21.3)
  line L615 (80.1273, 21.3) -> (82.2058, 20.1)
  line L616 (82.2058, 20.1) -> (84.2842, 21.3)
  line L617 (84.2842, 21.3) -> (84.2842, 23.7)
  line L618 (89.4804, 23.7) -> (87.4019, 24.9)
  line L619 (87.4019, 24.9) -> (85.3235, 23.7)
  line L620 (85.3235, 23.7) -> (85.3235, 21.3)
  line L621 (85.3235, 21.3) -> (87.4019, 20.1)
  line L622 (87.4019, 20.1) -> (89.4804, 21.3)
  line L623 (89.4804, 21.3) -> (89.4804, 23.7)
  line L624 (94.6765, 23.7) -> (92.5981, 24.9)
  line L625 (92.5981, 24.9) -> (90.5196, 23.7)
  line L626 (90.5196, 23.7) -> (90.5196, 21.3)
  line L627 (90.5196, 21.3) -> (92.5981, 20.1)
  line L628 (92.5981, 20.1) -> (94.6765, 21.3)
  line L629 (94.6765, 21.3) -> (94.6765, 23.7)
  line L630 (99.8727, 23.7) -> (97.7942, 24.9)
  line L631 (97.7942, 24.9) -> (95.7158, 23.7)
  line L632 (95.7158, 23.7) -> (95.7158, 21.3)
  line L633 (95.7158, 21.3) -> (97.7942, 20.1)
  line L634 (97.7942, 20.1) -> (99.8727, 21.3)
  line L635 (99.8727, 21.3) -> (99.8727, 23.7)
  line L636 (105.0688, 23.7) -> (102.9904, 24.9)
  line L637 (102.9904, 24.9) -> (100.9119, 23.7)
  line L638 (100.9119, 23.7) -> (100.9119, 21.3)
  line L639 (100.9119, 21.3) -> (102.9904, 20.1)
  line L640 (102.9904, 20.1) -> (105.0688, 21.3)
  line L641 (105.0688, 21.3) -> (105.0688, 23.7)
  line L642 (110.265, 23.7) -> (108.1865, 24.9)
  line L643 (108.1865, 24.9) -> (106.1081, 23.7)
  line L644 (106.1081, 23.7) -> (106.1081, 21.3)
  line L645 (106.1081, 21.3) -> (108.1865, 20.1)
  line L646 (108.1865, 20.1) -> (110.265, 21.3)
  line L647 (110.265, 21.3) -> (110.265, 23.7)
  line L648 (81.6862, 28.2) -> (79.6077, 29.4)
  line L649 (79.6077, 29.4) -> (77.5292, 28.2)
  line L650 (77.5292, 28.2) -> (77.5292, 25.8)
  line L651 (77.5292, 25.8) -> (79.6077, 24.6)
  line L652 (79.6077, 24.6) -> (81.6862, 25.8)
  line L653 (81.6862, 25.8) -> (81.6862, 28.2)
  line L654 (86.8823, 28.2) -> (84.8038, 29.4)
  line L655 (84.8038, 29.4) -> (82.7254, 28.2)
  line L656 (82.7254, 28.2) -> (82.7254, 25.8)
  line L657 (82.7254, 25.8) -> (84.8038, 24.6)
  line L658 (84.8038, 24.6) -> (86.8823, 25.8)
  line L659 (86.8823, 25.8) -> (86.8823, 28.2)
  line L660 (92.0785, 28.2) -> (90, 29.4)
  line L661 (90, 29.4) -> (87.9215, 28.2)
  line L662 (87.9215, 28.2) -> (87.9215, 25.8)
  line L663 (87.9215, 25.8) -> (90, 24.6)
  line L664 (90, 24.6) -> (92.0785, 25.8)
  line L665 (92.0785, 25.8) -> (92.0785, 28.2)
  line L666 (97.2746, 28.2) -> (95.1962, 29.4)
  line L667 (95.1962, 29.4) -> (93.1177, 28.2)
  line L668 (93.1177, 28.2) -> (93.1177, 25.8)
  line L669 (93.1177, 25.8) -> (95.1962, 24.6)
  line L670 (95.1962, 24.6) -> (97.2746, 25.8)
  line L671 (97.2746, 25.8) -> (97.2746, 28.2)
  line L672 (102.4708, 28.2) -> (100.3923, 29.4)
  line L673 (100.3923, 29.4) -> (98.3138, 28.2)
  line L674 (98.3138, 28.2) -> (98.3138, 25.8)
  line L675 (98.3138, 25.8) -> (100.3923, 24.6)
  line L676 (100.3923, 24.6) -> (102.4708, 25.8)
  line L677 (102.4708, 25.8) -> (102.4708, 28.2)
extrude "HexCut" cut sketch "HexGrid" along normal mid plane 10 bodies 2
named bodies: "Shell", "Lid"
